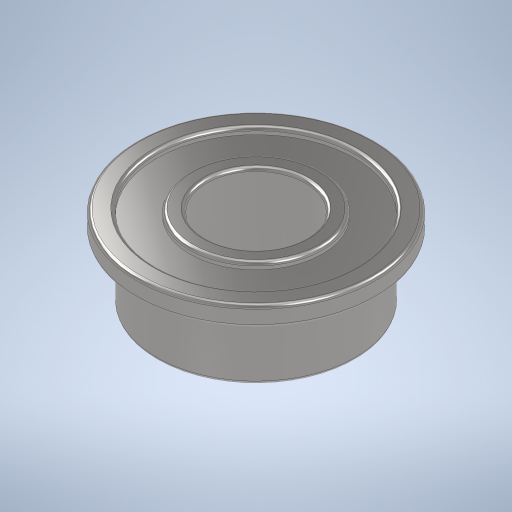
# Autodesk Inventor part: Bearing36
Saved by Autodesk Inventor 2024.3 (Build 283343010, 343A)
## iProperties
Created: 2025-12-01
Part Number: Bearing36
Material: ステンレス鋼
Document SubType Name: Modeling
Designer: kshau
Density: 8 g/cm^3
Appearance: 半つや出し
Author: kshau
Autodesk Inventor part; units mm, degrees
ref_plane "YZ Plane" through (0, 0, 0) normal (1, 0, 0) x (0, 1, 0)
ref_plane "XZ Plane" through (0, 0, 0) normal (0, 1, 0) x (-1, 0, 0)
ref_plane "XY Plane" through (0, 0, 0) normal (0, 0, 1) x (1, 0, 0)
sketch "スケッチ1" plane through (0, 0, 0) normal (0, 1, 0) x (-1, 0, 0)
  circle A0 centre (0, 0) radius 3.6
  dimension "d0" = 7.2
  constraints: 1 centre point, 1 coincident
  measures "d0" diameter of A0
extrude "押し出し1" add sketch "スケッチ1" along normal blind 0.6
sketch "スケッチ2" plane through (0, 0, 0) normal (0, -1, 0) x (1, 0, 0)
  circle A0 centre (0, 0) radius 3
  dimension "d3" = 6
  constraints: 1 centre point, 1 coincident
  measures "d3" diameter of A0
extrude "押し出し2" add sketch "スケッチ2" along normal blind 1.9
sketch "スケッチ3" plane through (0, -1.9, 0) normal (0, -1, 0) x (1, 0, 0)
  point P0 (0, 0)
  point P1 (0, 0)
  constraints: 1 coincident
hole "穴1" at (0, -1.9, 0) direction (0, 1, 0) diameter 3 end through all
sketch "スケッチ4" plane through (0, 0.6, 0) normal (0, 1, 0) x (1, 0, 0)
  circle A0 centre (0, 0) radius 2
  circle A1 centre (0, 0) radius 3
  dimension "d13" = 4
  dimension "d14" = 6
  constraints: 2 centre point, 2 coincident
  measures "d13" diameter of A0
  measures "d14" diameter of A1
extrude "押し出し3" cut sketch "スケッチ4" against normal blind 0.2
sketch "スケッチ5" plane through (0, -1.9, 0) normal (0, -1, 0) x (1, 0, 0)
  circle A0 centre (0, 0) radius 2
  circle A1 centre (0, 0) radius 2.5
  dimension "d18" = 4
  dimension "d19" = 5
  constraints: 2 centre point, 2 coincident
  measures "d18" diameter of A0
  measures "d19" diameter of A1
extrude "押し出し4" cut sketch "スケッチ5" against normal blind 0.2
fillet "フィレット2" radius 0.1 10 edges at (-3, -1.9, 0) (-2.5, -1.9, 0) (-2, -1.9, 0) (0, -1.9, 1.5) (-3, 0, 0) (3.6, 0, 0) (3.6, 0.6, 0) (-3, 0.6, 0) (-2, 0.6, 0) (0, 0.6, 1.5)
